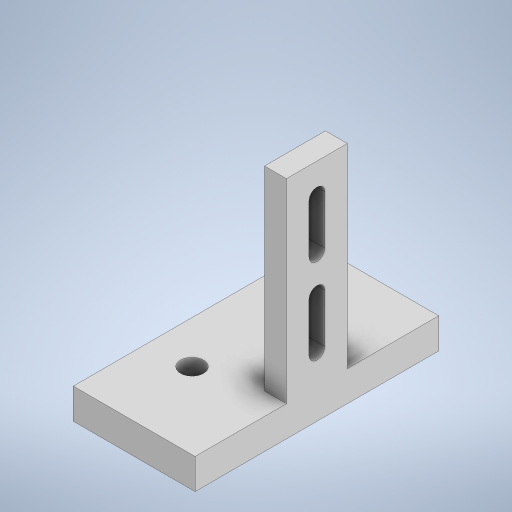
# Autodesk Inventor part: motor_u_adapter
Saved by Autodesk Inventor 2024 (Build 280153000, 153)
## iProperties
Created: 2023-11-06
Part Number: motor_u_adapter
Material: Generic
Document SubType Name: Modeling
Designer: dimademler
Density: 1 g/cm^3
Appearance: Default
Author: dimademler
Autodesk Inventor part; units mm, degrees
ref_plane "YZ Plane" through (0, 0, 0) normal (1, 0, 0) x (0, 1, 0)
ref_plane "XZ Plane" through (0, 0, 0) normal (0, 1, 0) x (-1, 0, 0)
ref_plane "XY Plane" through (0, 0, 0) normal (0, 0, 1) x (1, 0, 0)
sketch "Sketch15" plane through (0, 0, 0) normal (0, 1, 0) x (-1, 0, 0)
  line L0 (0, 0) -> (25.4, 0)
  line L1 (25.4, 0) -> (25.4, 50.8)
  line L2 (25.4, 50.8) -> (0, 50.8)
  line L3 (0, 50.8) -> (0, 0)
  dimension "d64" = 25.4
  dimension "d65" = 50.8
  constraints: 8 end point, 2 parallel, 1 horizontal, 1 perpendicular
  measures "d64" distance of L2.end L1.end
  measures "d65" distance of L1.end L0.end
extrude "Extrusion12" add sketch "Sketch15" along normal blind 6.35
sketch "Sketch17" plane through (0, 6.35, 0) normal (0, 1, 0) x (1, 0, 0)
  line L0 (-25.4, 0) -> (-25.4, -50.8) projected
  line L1 (-25.4, -50.8) -> (0, -50.8) projected
  line L2 (0, -50.8) -> (0, 0) projected
  line L3 (0, 0) -> (-25.4, 0) projected
  line L4 (0, -25.4) -> (0, -19.05)
  line L5 (0, -25.4) -> (0, -31.75)
  line L6 (0, -31.75) -> (-4.572, -31.75)
  line L7 (-4.572, -31.75) -> (0, -31.75)
  line L8 (0, -31.75) -> (0, -19.05)
  line L9 (0, -19.05) -> (-4.572, -19.05)
  line L10 (-4.572, -19.05) -> (-4.572, -31.75)
  dimension "d74" = 6.35
  dimension "d75" = 6.35
  dimension "d76" = 4.572
  constraints: 14 end point, 2 parallel, 2 perpendicular, 2 point on line, 1 horizontal, 1 midpoint
  measures "d74" distance of L4.start L4.end
  measures "d75" distance of L4.start L5.end
  measures "d76" distance of L5.end L6.end
extrude "Extrusion14" add sketch "Sketch17" along normal blind 40.64 contours L2 L6 L10 L9
sketch "Sketch18" plane through (-4.572, 6.35, 19.05) normal (-1, 0, 0) x (0, 0, 1)
  line L0 (12.7, 0) -> (0, 0) projected
  line L1 (12.7, 0) -> (12.7, 40.64) projected
  line L2 (0, 40.64) -> (12.7, 40.64) projected
  line L3 (0, 0) -> (0, 40.64) projected
  line L4 (0, 20.32) -> (12.7, 20.32) construction
  line L5 (6.35, 20.32) -> (6.35, 24.13) construction
  line L6 (6.35, 24.13) -> (6.35, 34.29) construction
  line L7 (8.001, 24.13) -> (8.001, 34.29)
  line L8 (4.699, 34.29) -> (4.699, 24.13)
  arc A0 (4.699, 24.13) -> (8.001, 24.13) centre (6.35, 24.13) ccw
  arc A1 (8.001, 34.29) -> (4.699, 34.29) centre (6.35, 34.29) ccw
  line L9 (8.001, 16.51) -> (8.001, 6.35)
  line L10 (4.699, 6.35) -> (4.699, 16.51)
  arc A2 (8.001, 16.51) -> (4.699, 16.51) centre (6.35, 16.51) ccw
  arc A3 (4.699, 6.35) -> (8.001, 6.35) centre (6.35, 6.35) ccw
  point P0 (-19.05, -6.35)
  point P1 (6.35, 29.21)
  dimension "d79" = 3.81
  dimension "d80" = 10.16
  dimension "d81" = 3.302
  constraints: 16 end point, 8 point on circle, 6 symmetric about line, 4 centre point, 4 midpoint, 4 tangent, 2 vertical, 1 parallel, 2 other
  measures "d79" distance of L5.start L5.end
  measures "d80" distance of L5.end L6.end
  measures "d81" diameter of A1
extrude "Extrusion15" cut sketch "Sketch18" against normal up to next contours A0 L8 A1 L7 | L9 A3 L10 A2
sketch "Sketch19" plane through (0, 6.35, 0) normal (0, 1, 0) x (1, 0, 0)
  line L0 (-4.572, -19.05) -> (0, -19.05) projected
  line L1 (0, -19.05) -> (0, 0) projected
  line L2 (0, 0) -> (-25.4, 0) projected
  line L3 (-25.4, 0) -> (-25.4, -50.8) projected
  line L4 (-25.4, -50.8) -> (0, -50.8) projected
  line L5 (0, -50.8) -> (0, -31.75) projected
  line L6 (0, -31.75) -> (-4.572, -31.75) projected
  line L7 (-4.572, -31.75) -> (-4.572, -19.05) projected
  line L8 (-25.4, -25.4) -> (0, -25.4) construction
  line L9 (0, -50.8) -> (0, 0) projected
  line L10 (-12.7, -25.4) -> (-16.51, -25.4)
  line L11 (-16.51, -25.4) -> (-16.51, -15.875) construction
  circle A0 centre (-16.51, -15.875) radius 2.413
  line L12 (-16.51, -25.4) -> (-16.51, -34.925) construction
  circle A1 centre (-16.51, -34.925) radius 2.413
  dimension "d84" = 3.81
  dimension "d85" = 9.525
  dimension "d86" = 4.826
  constraints: 8 end point, 3 midpoint, 2 centre point, 2 coincident, 2 symmetric about line, 1 perpendicular, 1 point on line, 1 other
  measures "d84" distance of L10.start L10.end
  measures "d85" distance of L10.end L11.end
  measures "d86" diameter of A0
extrude "Extrusion16" cut sketch "Sketch19" against normal up to next contours A0 | A1
equation "\"base_thickness\" = 6.35"
equation "\"motor_adapter_width\" = 19.05"
equation "\"d16\" = 0.5 * motor_adapter_width"
equation "\"motor_adapter_across\" = 21.59"
equation "\"motor_u_adapterthickness\" = 3.81"
body "Solid2"
